Autodesk Inventor part; units mm, degrees
(part 2 of 3)
  arc A175 (-37.2013, 68.5038) -> (-37.3635, 68.3097) centre (-36.1751, 67.4815) ccw
  line L41 (-37.3635, 68.3097) -> (-37.4284, 68.2167)
  line L42 (-37.4284, 68.2167) -> (-36.811, 67.6337)
  line L43 (-36.811, 67.6337) -> (-36.1936, 67.0508)
  line L44 (-36.1936, 67.0508) -> (-36.0674, 67.2032)
  arc A176 (-35.5543, 67.7509) -> (-36.0674, 67.2032) centre (-31.3354, 63.2844) ccw
  arc A177 (-34.9902, 68.2176) -> (-35.5543, 67.7509) centre (-31.7324, 63.7046) ccw
  arc A178 (-34.3783, 68.5998) -> (-34.9902, 68.2176) centre (-31.8294, 63.839) ccw
  arc A179 (-33.7228, 68.8958) -> (-34.3783, 68.5998) centre (-31.86, 63.8962) ccw
  arc A180 (-32.0401, 69.2429) -> (-33.7228, 68.8958) centre (-31.7577, 63.6217) ccw
  arc A181 (-30.349, 69.0602) -> (-32.0401, 69.2429) centre (-31.7686, 63.8379) ccw
  arc A182 (-28.7916, 68.3601) -> (-30.349, 69.0602) centre (-31.7807, 63.7933) ccw
  arc A183 (-27.4976, 67.2036) -> (-28.7916, 68.3601) centre (-31.976, 63.4949) ccw
  line L45 (-27.4976, 67.2036) -> (-27.3717, 67.0515)
  line L46 (-27.3717, 67.0515) -> (-26.7547, 67.6348)
  line L47 (-26.7547, 67.6348) -> (-26.1378, 68.218)
  line L48 (-26.1378, 68.218) -> (-26.2023, 68.3104)
  arc A184 (-26.2023, 68.3104) -> (-26.2473, 68.3665) centre (-26.6433, 68.0026) ccw
  arc A185 (-26.2473, 68.3665) -> (-26.3703, 68.4988) centre (-37.3359, 58.178) ccw
  arc A186 (-26.3703, 68.4988) -> (-26.5193, 68.6547) centre (-36.4537, 59.0082) ccw
  arc A187 (-26.5193, 68.6547) -> (-26.6838, 68.822) centre (-40.4031, 55.1733) ccw
  arc A188 (-26.6838, 68.822) -> (-27.1502, 69.256) centre (-32.5321, 63.0037) ccw
  arc A189 (-27.1502, 69.256) -> (-27.6227, 69.6261) centre (-31.3885, 64.3323) ccw
  arc A190 (-27.6227, 69.6261) -> (-28.1264, 69.9504) centre (-31.375, 64.3513) ccw
  arc A191 (-28.1264, 69.9504) -> (-28.687, 70.247) centre (-32.2022, 62.9256) ccw
  arc A192 (-28.687, 70.247) -> (-29.244, 70.4848) centre (-31.6549, 64.0655) ccw
  arc A193 (-29.244, 70.4848) -> (-29.8311, 70.6779) centre (-31.8578, 63.5254) ccw
  arc A194 (-29.8311, 70.6779) -> (-30.4329, 70.8217) centre (-31.863, 63.5069) ccw
  arc A195 (-30.4329, 70.8217) -> (-31.0343, 70.9122) centre (-31.7664, 64.0012) ccw
  arc A196 (-31.0343, 70.9122) -> (-31.3562, 70.9333) centre (-31.4614, 66.8798) ccw
  arc A197 (-31.3562, 70.9333) -> (-31.8226, 70.939) centre (-31.7967, 53.9604) ccw
  arc A198 (-31.8226, 70.939) -> (-32.2848, 70.9321) centre (-31.7963, 53.7113) ccw
  arc A199 (-32.2848, 70.9321) -> (-32.5832, 70.9098) centre (-32.1934, 67.7089) ccw
  arc A200 (-32.0904, 68.184) -> (-32.8869, 68.0454) centre (-31.5556, 62.7535) ccw
  arc A201 (-32.8869, 68.0454) -> (-33.6094, 67.7947) centre (-31.8192, 63.8013) ccw
  arc A202 (-33.6094, 67.7947) -> (-34.2629, 67.4283) centre (-31.8964, 63.9735) ccw
  arc A203 (-34.2629, 67.4283) -> (-34.854, 66.9451) centre (-31.7132, 63.7061) ccw
  arc A204 (-34.854, 66.9451) -> (-35.0438, 66.7534) centre (-30.2573, 62.2047) ccw
  arc A205 (-35.0438, 66.7534) -> (-35.2248, 66.5549) centre (-30.3374, 62.2808) ccw
  arc A206 (-35.2248, 66.5549) -> (-35.3825, 66.371) centre (-25.9009, 58.401) ccw
  arc A207 (-35.3825, 66.371) -> (-35.4014, 66.3193) centre (-35.321, 66.3193) ccw
  arc A208 (-35.4014, 66.3193) -> (-35.3918, 66.297) centre (-35.3708, 66.3193) ccw
  arc A209 (-35.3918, 66.297) -> (-34.7975, 65.7374) centre (1437.4655, 1629.9498) ccw
  arc A210 (-34.7975, 65.7374) -> (-34.211, 65.1858) centre (719.0411, 866.6564) ccw
  arc A211 (-34.211, 65.1858) -> (-34.1695, 65.1598) centre (-34.1239, 65.2785) ccw
  arc A212 (-34.1695, 65.1598) -> (-34.1552, 65.163) centre (-34.1647, 65.1721) ccw
  arc A213 (-34.1552, 65.163) -> (-34.1121, 65.2103) centre (-35.4224, 66.3612) ccw
  arc A214 (-34.1121, 65.2103) -> (-34.062, 65.2709) centre (-35.0787, 66.0593) ccw
  arc A215 (-34.062, 65.2709) -> (-34.0071, 65.3446) centre (-35.9526, 66.7371) ccw
  arc A216 (-33.6777, 65.7235) -> (-34.0071, 65.3446) centre (-31.8426, 63.7953) ccw
  arc A217 (-33.2793, 66.0389) -> (-33.6777, 65.7235) centre (-31.7523, 63.7004) ccw
  arc A218 (-32.8278, 66.2785) -> (-33.2793, 66.0389) centre (-31.7341, 63.6725) ccw
  arc A219 (-32.3411, 66.4325) -> (-32.8278, 66.2785) centre (-31.7393, 63.6849) ccw
  arc A220 (-32.0556, 66.4702) -> (-32.3411, 66.4325) centre (-31.9755, 64.7634) ccw
  arc A221 (-31.6858, 66.4725) -> (-32.0556, 66.4702) centre (-31.8417, 61.911) ccw
  arc A222 (-31.3168, 66.4449) -> (-31.6858, 66.4725) centre (-31.8418, 61.9075) ccw
  arc A223 (-31.0333, 66.3878) -> (-31.3168, 66.4449) centre (-31.5158, 64.7246) ccw
  arc A224 (-30.6006, 66.2181) -> (-31.0333, 66.3878) centre (-31.743, 63.9414) ccw
  arc A225 (-30.1846, 65.966) -> (-30.6006, 66.2181) centre (-31.9687, 63.4917) ccw
  arc A226 (-29.8154, 65.652) -> (-30.1846, 65.966) centre (-31.9569, 63.5081) ccw
  arc A227 (-29.5219, 65.298) -> (-29.8154, 65.652) centre (-31.554, 63.9115) ccw
  arc A228 (-29.5219, 65.298) -> (-29.4814, 65.242) centre (-28.4557, 66.0255) ccw
  arc A229 (-29.4814, 65.242) -> (-29.4433, 65.1963) centre (-28.9168, 65.6733) ccw
  arc A230 (-29.4433, 65.1963) -> (-29.4105, 65.1624) centre (-28.9075, 65.6817) ccw
  arc A231 (-29.4105, 65.1624) -> (-29.3963, 65.1594) centre (-29.4011, 65.1721) ccw
  arc A232 (-29.3963, 65.1594) -> (-29.3562, 65.1846) centre (-29.44, 65.2739) ccw
  arc A233 (-29.3562, 65.1846) -> (-28.7682, 65.7366) centre (-840.8345, 930.1184) ccw
  arc A234 (-28.7682, 65.7366) -> (-28.1727, 66.2963) centre (-1600.6595, 1738.8944) ccw
  arc A235 (-28.1727, 66.2963) -> (-28.1634, 66.3178) centre (-28.1929, 66.3178) ccw
  arc A236 (-28.1634, 66.3178) -> (-28.1663, 66.3266) centre (-28.1782, 66.3178) ccw
  arc A237 (-28.1663, 66.3266) -> (-28.2084, 66.3834) centre (-38.1616, 58.9544) ccw
  arc A238 (-28.2084, 66.3834) -> (-28.258, 66.4485) centre (-31.6783, 63.7935) ccw
  arc A239 (-28.258, 66.4485) -> (-28.3168, 66.5233) centre (-34.5032, 61.6007) ccw
  arc A240 (-28.3168, 66.5233) -> (-28.6224, 66.8616) centre (-31.1638, 64.2579) ccw
  arc A241 (-28.6224, 66.8616) -> (-29.0001, 67.1976) centre (-32.4574, 62.9327) ccw
  arc A242 (-29.0001, 67.1976) -> (-29.4081, 67.4984) centre (-32.4734, 62.9129) ccw
  arc A243 (-29.4081, 67.4984) -> (-29.8056, 67.7302) centre (-31.4926, 64.3801) ccw
  arc A244 (-29.8056, 67.7302) -> (-30.0614, 67.8432) centre (-31.0503, 65.2584) ccw
  arc A245 (-30.0614, 67.8432) -> (-30.3939, 67.9608) centre (-32.5323, 61.3851) ccw
  arc A246 (-30.3939, 67.9608) -> (-30.7335, 68.0617) centre (-32.5419, 61.3556) ccw
  arc A247 (-30.7335, 68.0617) -> (-31.0124, 68.1226) centre (-31.5028, 65.209) ccw
  arc A248 (-31.0124, 68.1226) -> (-31.2629, 68.1554) centre (-31.5838, 64.7277) ccw
  arc A249 (-31.2629, 68.1554) -> (-31.5824, 68.1794) centre (-32.0821, 59.4058) ccw
  arc A250 (-31.5824, 68.1794) -> (-31.8907, 68.1916) centre (-32.0866, 59.3265) ccw
  arc A251 (-31.8907, 68.1916) -> (-32.0904, 68.184) centre (-31.9274, 66.5294) ccw
  arc A252 (-32.1366, 65.3865) -> (-32.5528, 65.1937) centre (-31.7549, 64.017) ccw
  arc A253 (-32.5528, 65.1937) -> (-32.8895, 64.8772) centre (-31.7317, 63.9828) ccw
  arc A254 (-32.8895, 64.8772) -> (-33.1084, 64.4743) centre (-31.7513, 63.998) ccw
  arc A255 (-33.1084, 64.4743) -> (-33.1834, 64.0313) centre (-31.8538, 64.0339) ccw
  arc A256 (-33.1834, 64.0313) -> (-33.0398, 63.4203) centre (-31.8003, 64.0341) ccw
  arc A257 (-33.0398, 63.4203) -> (-32.6401, 62.9292) centre (-31.759, 64.0545) ccw
  arc A258 (-32.6401, 62.9292) -> (-32.07, 62.6613) centre (-31.7694, 64.0412) ccw
  arc A259 (-32.07, 62.6613) -> (-31.4495, 62.6738) centre (-31.7859, 63.9654) ccw
  arc A260 (-31.4495, 62.6738) -> (-31.0909, 62.817) centre (-31.839, 64.1692) ccw
  arc A261 (-31.0909, 62.817) -> (-30.7938, 63.0407) centre (-31.7358, 63.9827) ccw
  arc A262 (-30.7938, 63.0407) -> (-30.5702, 63.3378) centre (-31.7358, 63.9827) ccw
  arc A263 (-30.5702, 63.3378) -> (-30.4269, 63.6964) centre (-31.9224, 64.0859) ccw
  arc A264 (-30.4269, 63.6964) -> (-30.4151, 64.3239) centre (-31.7256, 64.0347) ccw
  arc A265 (-30.4151, 64.3239) -> (-30.6888, 64.8964) centre (-31.7815, 64.0223) ccw
  arc A266 (-30.6888, 64.8964) -> (-31.1897, 65.2927) centre (-31.7983, 64.0089) ccw
  arc A267 (-31.1897, 65.2927) -> (-31.8119, 65.4279) centre (-31.7912, 64.0239) ccw
  arc A268 (-31.8119, 65.4279) -> (-31.8933, 65.424) centre (-31.7935, 64.1823) ccw
  arc A269 (-31.8933, 65.424) -> (-31.984, 65.4146) centre (-31.7364, 63.4723) ccw
  arc A270 (-31.984, 65.4146) -> (-32.0702, 65.4015) centre (-31.75, 63.5786) ccw
  arc A271 (-32.0702, 65.4015) -> (-32.1366, 65.3865) centre (-31.95, 64.7171) ccw
  arc A272 (-30.9168, 15.2189) -> (-29.3545, 15.4735) centre (-31.794, 25.5192) ccw
  arc A273 (-29.3545, 15.4735) -> (-27.8672, 15.9622) centre (-31.6889, 25.0867) ccw
  arc A274 (-27.8672, 15.9622) -> (-26.477, 16.6788) centre (-31.6817, 25.0694) ccw
  arc A275 (-26.477, 16.6788) -> (-25.2034, 17.6119) centre (-31.8789, 25.3873) ccw
  arc A276 (-25.2034, 17.6119) -> (-24.9272, 17.861) centre (-30.1736, 23.401) ccw
  arc A277 (-24.9272, 17.861) -> (-24.6106, 18.1697) centre (-35.3442, 28.861) ccw
  arc A278 (-24.6106, 18.1697) -> (-24.3181, 18.4718) centre (-35.0871, 28.6048) ccw
  arc A279 (-24.3181, 18.4718) -> (-24.1302, 18.6893) centre (-26.7779, 20.7864) ccw
  line L49 (-24.1302, 18.6893) -> (-24.0364, 18.8078)
  line L50 (-24.0364, 18.8078) -> (-24.6584, 19.3804)
  line L51 (-24.6584, 19.3804) -> (-25.2804, 19.9531)
  line L52 (-25.2804, 19.9531) -> (-25.4467, 19.7631)
  arc A280 (-26.4222, 18.8133) -> (-25.4467, 19.7631) centre (-31.8805, 25.3952) ccw
  arc A281 (-27.5365, 18.0299) -> (-26.4222, 18.8133) centre (-31.8906, 25.4074) ccw
  arc A282 (-28.7501, 17.4395) -> (-27.5365, 18.0299) centre (-31.81, 25.2709) ccw
  arc A283 (-30.0209, 17.0635) -> (-28.7501, 17.4395) centre (-31.5963, 24.724) ccw
  arc A284 (-30.8588, 16.936) -> (-30.0209, 17.0635) centre (-31.6693, 25.079) ccw
  arc A285 (-31.7176, 16.8933) -> (-30.8588, 16.936) centre (-31.7176, 25.5643) ccw
  arc A286 (-32.5765, 16.936) -> (-31.7176, 16.8933) centre (-31.7176, 25.5643) ccw
  arc A287 (-33.4143, 17.0635) -> (-32.5765, 16.936) centre (-31.7659, 25.079) ccw
  arc A288 (-34.6853, 17.439) -> (-33.4143, 17.0635) centre (-31.8322, 24.7569) ccw
  arc A289 (-35.8956, 18.0273) -> (-34.6853, 17.439) centre (-31.653, 25.2164) ccw
  arc A290 (-37.0081, 18.8098) -> (-35.8956, 18.0273) centre (-31.5598, 25.3743) ccw
  arc A291 (-37.9883, 19.7628) -> (-37.0081, 18.8098) centre (-31.4492, 25.5076) ccw
  line L53 (-37.9883, 19.7628) -> (-38.1548, 19.9524)
  line L54 (-38.1548, 19.9524) -> (-38.7772, 19.3805)
  line L55 (-38.7772, 19.3805) -> (-39.3995, 18.8086)
  line L56 (-39.3995, 18.8086) -> (-39.3018, 18.6827)
  arc A292 (-39.3018, 18.6827) -> (-39.0982, 18.4502) centre (-37.247, 20.277) ccw
  arc A293 (-39.0982, 18.4502) -> (-38.6947, 18.0503) centre (-20.8164, 36.4914) ccw
  arc A294 (-38.6947, 18.0503) -> (-38.2739, 17.6523) centre (-22.4071, 34.8506) ccw
  arc A295 (-38.2739, 17.6523) -> (-37.97, 17.3915) centre (-34.4969, 21.7463) ccw
  arc A296 (-37.97, 17.3915) -> (-36.7254, 16.5398) centre (-31.5357, 25.4591) ccw
  arc A297 (-36.7254, 16.5398) -> (-35.3826, 15.8887) centre (-31.7481, 25.0939) ccw
  arc A298 (-35.3826, 15.8887) -> (-33.9556, 15.4462) centre (-31.7395, 25.1157) ccw
  arc A299 (-33.9556, 15.4462) -> (-32.4601, 15.2161) centre (-31.6251, 25.6151) ccw
  arc A300 (-32.4601, 15.2161) -> (-32.0962, 15.1956) centre (-31.8541, 22.7628) ccw
  arc A301 (-32.0962, 15.1956) -> (-31.6859, 15.1895) centre (-31.708, 27.3292) ccw
  arc A302 (-31.6859, 15.1895) -> (-31.2769, 15.1971) centre (-31.7079, 27.2755) ccw
  arc A303 (-31.2769, 15.1971) -> (-30.9168, 15.2189) centre (-31.538, 22.5135) ccw
  arc A304 (-30.9168, 17.9902) -> (-29.9577, 18.169) centre (-31.8527, 25.6751) ccw
  arc A305 (-29.9577, 18.169) -> (-29.0477, 18.4646) centre (-31.7105, 25.112) ccw
  arc A306 (-29.0477, 18.4646) -> (-28.1832, 18.8798) centre (-31.724, 25.1455) ccw
  arc A307 (-28.1832, 18.8798) -> (-27.3594, 19.4152) centre (-32.0807, 25.7768) ccw
  arc A308 (-27.3594, 19.4152) -> (-27.0939, 19.6338) centre (-29.3965, 22.1601) ccw
  arc A309 (-27.0939, 19.6338) -> (-26.6906, 20.0113) centre (-41.2454, 35.1596) ccw
  arc A310 (-26.6906, 20.0113) -> (-26.2987, 20.3962) centre (-44.0969, 38.1275) ccw
  arc A311 (-26.2987, 20.3962) -> (-26.1365, 20.5903) centre (-27.3249, 21.4185) ccw
  line L57 (-26.1365, 20.5903) -> (-26.0716, 20.6833)
  line L58 (-26.0716, 20.6833) -> (-26.689, 21.2663)
  line L59 (-26.689, 21.2663) -> (-27.3064, 21.8492)
  line L60 (-27.3064, 21.8492) -> (-27.4326, 21.6968)
  arc A312 (-27.9457, 21.1491) -> (-27.4326, 21.6968) centre (-32.1646, 25.6156) ccw
  arc A313 (-28.5098, 20.6824) -> (-27.9457, 21.1491) centre (-31.7676, 25.1954) ccw
  arc A314 (-29.1217, 20.3002) -> (-28.5098, 20.6824) centre (-31.6706, 25.061) ccw
  arc A315 (-29.7772, 20.0042) -> (-29.1217, 20.3002) centre (-31.64, 25.0038) ccw
  arc A316 (-31.4599, 19.6571) -> (-29.7772, 20.0042) centre (-31.7423, 25.2783) ccw
  arc A317 (-33.151, 19.8398) -> (-31.4599, 19.6571) centre (-31.7314, 25.0621) ccw
  arc A318 (-34.7084, 20.5399) -> (-33.151, 19.8398) centre (-31.7193, 25.1067) ccw
  arc A319 (-36.0024, 21.6964) -> (-34.7084, 20.5399) centre (-31.524, 25.4051) ccw
  line L61 (-36.0024, 21.6964) -> (-36.1283, 21.8485)
  line L62 (-36.1283, 21.8485) -> (-36.7453, 21.2652)
  line L63 (-36.7453, 21.2652) -> (-37.3622, 20.682)
  line L64 (-37.3622, 20.682) -> (-37.2977, 20.5896)
  arc A320 (-37.2977, 20.5896) -> (-37.2527, 20.5335) centre (-36.8567, 20.8974) ccw
  arc A321 (-37.2527, 20.5335) -> (-37.1297, 20.4012) centre (-26.1641, 30.722) ccw
  arc A322 (-37.1297, 20.4012) -> (-36.9807, 20.2453) centre (-27.0463, 29.8918) ccw
  arc A323 (-36.9807, 20.2453) -> (-36.8162, 20.078) centre (-23.0969, 33.7267) ccw
  arc A324 (-36.8162, 20.078) -> (-36.3498, 19.644) centre (-30.9679, 25.8963) ccw
  arc A325 (-36.3498, 19.644) -> (-35.8773, 19.2739) centre (-32.1115, 24.5677) ccw
  arc A326 (-35.8773, 19.2739) -> (-35.3736, 18.9496) centre (-32.125, 24.5487) ccw
  arc A327 (-35.3736, 18.9496) -> (-34.813, 18.653) centre (-31.2978, 25.9744) ccw
  arc A328 (-34.813, 18.653) -> (-34.256, 18.4152) centre (-31.8451, 24.8345) ccw
  arc A329 (-34.256, 18.4152) -> (-33.6689, 18.2221) centre (-31.6422, 25.3746) ccw
  arc A330 (-33.6689, 18.2221) -> (-33.0671, 18.0783) centre (-31.637, 25.3931) ccw
  arc A331 (-33.0671, 18.0783) -> (-32.4657, 17.9878) centre (-31.7336, 24.8988) ccw
  arc A332 (-32.4657, 17.9878) -> (-32.1438, 17.9667) centre (-32.0386, 22.0202) ccw
  arc A333 (-32.1438, 17.9667) -> (-31.6774, 17.961) centre (-31.7033, 34.9396) ccw
  arc A334 (-31.6774, 17.961) -> (-31.2152, 17.9679) centre (-31.7037, 35.1887) ccw
  arc A335 (-31.2152, 17.9679) -> (-30.9168, 17.9902) centre (-31.3066, 21.1911) ccw
  arc A336 (-31.4096, 20.716) -> (-30.6131, 20.8546) centre (-31.9444, 26.1465) ccw
  arc A337 (-30.6131, 20.8546) -> (-29.8906, 21.1053) centre (-31.6808, 25.0987) ccw
  arc A338 (-29.8906, 21.1053) -> (-29.2371, 21.4717) centre (-31.6036, 24.9265) ccw
  arc A339 (-29.2371, 21.4717) -> (-28.646, 21.9549) centre (-31.7868, 25.1939) ccw
  arc A340 (-28.646, 21.9549) -> (-28.4562, 22.1466) centre (-33.2427, 26.6953) ccw
  arc A341 (-28.4562, 22.1466) -> (-28.2752, 22.3451) centre (-33.1626, 26.6192) ccw
  arc A342 (-28.2752, 22.3451) -> (-28.1175, 22.529) centre (-37.5991, 30.499) ccw
  arc A343 (-28.1175, 22.529) -> (-28.0986, 22.5807) centre (-28.179, 22.5807) ccw
  arc A344 (-28.0986, 22.5807) -> (-28.1082, 22.603) centre (-28.1292, 22.5807) ccw
  arc A345 (-28.1082, 22.603) -> (-28.7025, 23.1626) centre (-1500.9655, -1541.0498) ccw
  arc A346 (-28.7025, 23.1626) -> (-29.289, 23.7142) centre (-782.5411, -777.7564) ccw
  arc A347 (-29.289, 23.7142) -> (-29.3305, 23.7402) centre (-29.3761, 23.6215) ccw
  arc A348 (-29.3305, 23.7402) -> (-29.3448, 23.737) centre (-29.3353, 23.7279) ccw
  arc A349 (-29.3448, 23.737) -> (-29.3879, 23.6897) centre (-28.0776, 22.5388) ccw
  arc A350 (-29.3879, 23.6897) -> (-29.438, 23.6291) centre (-28.4213, 22.8407) ccw
  arc A351 (-29.438, 23.6291) -> (-29.4929, 23.5554) centre (-27.5474, 22.1629) ccw
  arc A352 (-29.8223, 23.1765) -> (-29.4929, 23.5554) centre (-31.6574, 25.1047) ccw
  arc A353 (-30.2207, 22.8611) -> (-29.8223, 23.1765) centre (-31.7477, 25.1996) ccw
  arc A354 (-30.6722, 22.6215) -> (-30.2207, 22.8611) centre (-31.7659, 25.2275) ccw
  arc A355 (-31.1589, 22.4675) -> (-30.6722, 22.6215) centre (-31.7607, 25.2151) ccw
  arc A356 (-31.4444, 22.4298) -> (-31.1589, 22.4675) centre (-31.5245, 24.1366) ccw
  arc A357 (-31.8142, 22.4275) -> (-31.4444, 22.4298) centre (-31.6583, 26.989) ccw
  arc A358 (-32.1832, 22.4551) -> (-31.8142, 22.4275) centre (-31.6582, 26.9925) ccw
  arc A359 (-32.4667, 22.5122) -> (-32.1832, 22.4551) centre (-31.9842, 24.1754) ccw
  arc A360 (-32.8994, 22.6819) -> (-32.4667, 22.5122) centre (-31.757, 24.9586) ccw
  arc A361 (-33.3154, 22.934) -> (-32.8994, 22.6819) centre (-31.5313, 25.4083) ccw
  arc A362 (-33.6846, 23.248) -> (-33.3154, 22.934) centre (-31.5431, 25.3919) ccw
  arc A363 (-33.9781, 23.602) -> (-33.6846, 23.248) centre (-31.946, 24.9885) ccw
  arc A364 (-33.9781, 23.602) -> (-34.0186, 23.658) centre (-35.0443, 22.8745) ccw
  arc A365 (-34.0186, 23.658) -> (-34.0567, 23.7037) centre (-34.5832, 23.2267) ccw
  arc A366 (-34.0567, 23.7037) -> (-34.0895, 23.7376) centre (-34.5925, 23.2183) ccw
  arc A367 (-34.0895, 23.7376) -> (-34.1037, 23.7406) centre (-34.0989, 23.7279) ccw
  arc A368 (-34.1037, 23.7406) -> (-34.1438, 23.7154) centre (-34.06, 23.6261) ccw
  arc A369 (-34.1438, 23.7154) -> (-34.7318, 23.1634) centre (777.3345, -841.2184) ccw
  arc A370 (-34.7318, 23.1634) -> (-35.3273, 22.6037) centre (1537.1595, -1649.9944) ccw
  arc A371 (-35.3273, 22.6037) -> (-35.3366, 22.5822) centre (-35.3071, 22.5822) ccw
  arc A372 (-35.3366, 22.5822) -> (-35.3337, 22.5734) centre (-35.3218, 22.5822) ccw
  arc A373 (-35.3337, 22.5734) -> (-35.2916, 22.5166) centre (-25.3384, 29.9456) ccw
  arc A374 (-35.2916, 22.5166) -> (-35.242, 22.4515) centre (-31.8217, 25.1065) ccw
  arc A375 (-35.242, 22.4515) -> (-35.1832, 22.3767) centre (-28.9968, 27.2993) ccw
  arc A376 (-35.1832, 22.3767) -> (-34.8776, 22.0384) centre (-32.3362, 24.6421) ccw
  arc A377 (-34.8776, 22.0384) -> (-34.4999, 21.7024) centre (-31.0426, 25.9673) ccw
  arc A378 (-34.4999, 21.7024) -> (-34.0919, 21.4016) centre (-31.0266, 25.9871) ccw
  arc A379 (-34.0919, 21.4016) -> (-33.6944, 21.1698) centre (-32.0074, 24.5199) ccw
  arc A380 (-33.6944, 21.1698) -> (-33.4386, 21.0568) centre (-32.4497, 23.6416) ccw
  arc A381 (-33.4386, 21.0568) -> (-33.1061, 20.9392) centre (-30.9677, 27.5149) ccw
  arc A382 (-33.1061, 20.9392) -> (-32.7665, 20.8383) centre (-30.9581, 27.5444) ccw
  arc A383 (-32.7665, 20.8383) -> (-32.4876, 20.7774) centre (-31.9972, 23.691) ccw
  arc A384 (-32.4876, 20.7774) -> (-32.2371, 20.7446) centre (-31.9162, 24.1723) ccw
  arc A385 (-32.2371, 20.7446) -> (-31.9176, 20.7206) centre (-31.4179, 29.4942) ccw
  arc A386 (-31.9176, 20.7206) -> (-31.6093, 20.7084) centre (-31.4134, 29.5735) ccw
  arc A387 (-31.6093, 20.7084) -> (-31.4096, 20.716) centre (-31.5726, 22.3706) ccw
  arc A388 (-31.3634, 23.5135) -> (-30.9472, 23.7063) centre (-31.7451, 24.883) ccw
  arc A389 (-30.9472, 23.7063) -> (-30.6105, 24.0228) centre (-31.7683, 24.9172) ccw
  arc A390 (-30.6105, 24.0228) -> (-30.3916, 24.4257) centre (-31.7487, 24.902) ccw
  arc A391 (-30.3916, 24.4257) -> (-30.3166, 24.8687) centre (-31.6462, 24.8661) ccw
  arc A392 (-30.3166, 24.8687) -> (-30.4602, 25.4797) centre (-31.6997, 24.8659) ccw
  arc A393 (-30.4602, 25.4797) -> (-30.8599, 25.9708) centre (-31.741, 24.8455) ccw
  arc A394 (-30.8599, 25.9708) -> (-31.43, 26.2387) centre (-31.7306, 24.8588) ccw
  arc A395 (-31.43, 26.2387) -> (-32.0505, 26.2262) centre (-31.7141, 24.9346) ccw
  arc A396 (-32.0505, 26.2262) -> (-32.4091, 26.083) centre (-31.661, 24.7308) ccw
  arc A397 (-32.4091, 26.083) -> (-32.7062, 25.8593) centre (-31.7642, 24.9173) ccw
  arc A398 (-32.7062, 25.8593) -> (-32.9298, 25.5622) centre (-31.7642, 24.9173) ccw
  arc A399 (-32.9298, 25.5622) -> (-33.0731, 25.2036) centre (-31.5776, 24.8141) ccw
  arc A400 (-33.0731, 25.2036) -> (-33.0849, 24.5761) centre (-31.7744, 24.8653) ccw
  arc A401 (-33.0849, 24.5761) -> (-32.8112, 24.0036) centre (-31.7185, 24.8777) ccw
  arc A402 (-32.8112, 24.0036) -> (-32.3103, 23.6073) centre (-31.7017, 24.8911) ccw
  arc A403 (-32.3103, 23.6073) -> (-31.6881, 23.4721) centre (-31.7088, 24.8761) ccw
  arc A404 (-31.6881, 23.4721) -> (-31.6067, 23.476) centre (-31.7065, 24.7177) ccw
  arc A405 (-31.6067, 23.476) -> (-31.516, 23.4854) centre (-31.7636, 25.4277) ccw
  arc A406 (-31.516, 23.4854) -> (-31.4298, 23.4985) centre (-31.75, 25.3214) ccw
  arc A407 (-31.4298, 23.4985) -> (-31.3634, 23.5135) centre (-31.55, 24.1829) ccw
  arc A408 (-54.2587, 71.8195) -> (-55.2164, 71.6633) centre (-53.721, 65.5053) ccw
  arc A409 (-55.2164, 71.6633) -> (-56.1281, 71.3638) centre (-53.7854, 65.7705) ccw
  arc A410 (-56.1281, 71.3638) -> (-56.9803, 70.9245) centre (-53.7898, 65.7811) ccw
  arc A411 (-56.9803, 70.9245) -> (-57.761, 70.3525) centre (-53.6689, 65.5862) ccw
  arc A412 (-57.761, 70.3525) -> (-57.9303, 70.1998) centre (-54.7143, 66.8038) ccw
  arc A413 (-57.9303, 70.1998) -> (-58.1244, 70.0106) centre (-51.5447, 63.4568) ccw
  arc A414 (-58.1244, 70.0106) -> (-58.3037, 69.8254) centre (-51.7023, 63.6139) ccw
  arc A415 (-58.3037, 69.8254) -> (-58.4189, 69.6921) centre (-56.7958, 68.4066) ccw
  line L65 (-58.4189, 69.6921) -> (-58.4764, 69.6194)
  line L66 (-58.4764, 69.6194) -> (-58.0951, 69.2684)
  line L67 (-58.0951, 69.2684) -> (-57.7138, 68.9174)
  line L68 (-57.7138, 68.9174) -> (-57.6118, 69.0338)
  arc A416 (-57.0139, 69.616) -> (-57.6118, 69.0338) centre (-53.6679, 65.5813) ccw
  arc A417 (-56.3308, 70.0963) -> (-57.0139, 69.616) centre (-53.6618, 65.5739) ccw
  arc A418 (-55.5869, 70.4582) -> (-56.3308, 70.0963) centre (-53.7111, 65.6576) ccw
  arc A419 (-54.8079, 70.6887) -> (-55.5869, 70.4582) centre (-53.8421, 65.9928) ccw
  arc A420 (-54.2943, 70.7669) -> (-54.8079, 70.6887) centre (-53.7974, 65.7752) ccw
  arc A421 (-53.7678, 70.793) -> (-54.2943, 70.7669) centre (-53.7678, 65.4777) ccw
  arc A422 (-53.2413, 70.7669) -> (-53.7678, 70.793) centre (-53.7678, 65.4777) ccw
  arc A423 (-52.7277, 70.6887) -> (-53.2413, 70.7669) centre (-53.7382, 65.7752) ccw
  arc A424 (-51.9486, 70.4585) -> (-52.7277, 70.6887) centre (-53.6976, 65.9726) ccw
  arc A425 (-51.2067, 70.0979) -> (-51.9486, 70.4585) centre (-53.8074, 65.6909) ccw
  arc A426 (-50.5247, 69.6182) -> (-51.2067, 70.0979) centre (-53.8645, 65.5942) ccw
  arc A427 (-49.9239, 69.034) -> (-50.5247, 69.6182) centre (-53.9323, 65.5125) ccw
  line L69 (-49.9239, 69.034) -> (-49.8218, 68.9178)
  line L70 (-49.8218, 68.9178) -> (-49.4403, 69.2684)
  line L71 (-49.4403, 69.2684) -> (-49.0588, 69.619)
  line L72 (-49.0588, 69.619) -> (-49.1187, 69.6961)
  arc A428 (-49.1187, 69.6961) -> (-49.2435, 69.8387) centre (-50.3783, 68.7188) ccw
  arc A429 (-49.2435, 69.8387) -> (-49.4908, 70.0838) centre (-60.4502, 58.7794) ccw
  arc A430 (-49.4908, 70.0838) -> (-49.7488, 70.3278) centre (-59.4752, 59.7852) ccw
  arc A431 (-49.7488, 70.3278) -> (-49.9351, 70.4876) centre (-52.0641, 67.8182) ccw
  arc A432 (-49.9351, 70.4876) -> (-50.698, 71.0097) centre (-53.8793, 65.5422) ccw
  arc A433 (-50.698, 71.0097) -> (-51.5212, 71.4089) centre (-53.7491, 65.766) ccw
  arc A434 (-51.5212, 71.4089) -> (-52.3959, 71.6801) centre (-53.7544, 65.7527) ccw
  arc A435 (-52.3959, 71.6801) -> (-53.3127, 71.8212) centre (-53.8245, 65.4466) ccw
  arc A436 (-53.3127, 71.8212) -> (-53.5357, 71.8337) centre (-53.6841, 67.195) ccw
  arc A437 (-53.5357, 71.8337) -> (-53.7872, 71.8375) centre (-53.7737, 64.3958) ccw
  arc A438 (-53.7872, 71.8375) -> (-54.0379, 71.8328) centre (-53.7737, 64.4287) ccw
  arc A439 (-54.0379, 71.8328) -> (-54.2587, 71.8195) centre (-53.8779, 67.3479) ccw
  arc A440 (-54.2587, 70.1206) -> (-54.8466, 70.011) centre (-53.685, 65.4098) ccw
  arc A441 (-54.8466, 70.011) -> (-55.4044, 69.8298) centre (-53.7721, 65.755) ccw
  arc A442 (-55.4044, 69.8298) -> (-55.9344, 69.5753) centre (-53.7639, 65.7344) ccw
  arc A443 (-55.9344, 69.5753) -> (-56.4394, 69.2471) centre (-53.5452, 65.3475) ccw
  arc A444 (-56.4394, 69.2471) -> (-56.6021, 69.1131) centre (-55.1906, 67.5645) ccw
  arc A445 (-56.6021, 69.1131) -> (-56.8494, 68.8817) centre (-47.9272, 59.5958) ccw
  arc A446 (-56.8494, 68.8817) -> (-57.0896, 68.6458) centre (-46.1793, 57.7765) ccw
  arc A447 (-57.0896, 68.6458) -> (-57.189, 68.5268) centre (-56.4605, 68.0191) ccw
  line L73 (-57.189, 68.5268) -> (-57.2288, 68.4697)
  line L74 (-57.2288, 68.4697) -> (-56.8503, 68.1124)
  line L75 (-56.8503, 68.1124) -> (-56.4719, 67.7551)
  line L76 (-56.4719, 67.7551) -> (-56.3945, 67.8485)
  arc A448 (-56.08, 68.1842) -> (-56.3945, 67.8485) centre (-53.4938, 65.4462) ccw
  arc A449 (-55.7342, 68.4703) -> (-56.08, 68.1842) centre (-53.7371, 65.7039) ccw
  arc A450 (-55.3591, 68.7046) -> (-55.7342, 68.4703) centre (-53.7966, 65.7862) ccw
  arc A451 (-54.9572, 68.886) -> (-55.3591, 68.7046) centre (-53.8154, 65.8213) ccw
  arc A452 (-53.9257, 69.0988) -> (-54.9572, 68.886) centre (-53.7527, 65.653) ccw
  arc A453 (-52.8891, 68.9868) -> (-53.9257, 69.0988) centre (-53.7593, 65.7856) ccw
  arc A454 (-51.9344, 68.5576) -> (-52.8891, 68.9868) centre (-53.7667, 65.7582) ccw
  arc A455 (-51.1412, 67.8487) -> (-51.9344, 68.5576) centre (-53.8865, 65.5753) ccw
  line L77 (-51.1412, 67.8487) -> (-51.064, 67.7555)
  line L78 (-51.064, 67.7555) -> (-50.6858, 68.113)
  line L79 (-50.6858, 68.113) -> (-50.3077, 68.4706)
  line L80 (-50.3077, 68.4706) -> (-50.3472, 68.5272)
  arc A456 (-50.3472, 68.5272) -> (-50.3748, 68.5616) centre (-50.6176, 68.3385) ccw
  arc A457 (-50.3748, 68.5616) -> (-50.4502, 68.6427) centre (-57.1721, 62.316) ccw
  arc A458 (-50.4502, 68.6427) -> (-50.5416, 68.7383) centre (-56.6313, 62.825) ccw
  arc A459 (-50.5416, 68.7383) -> (-50.6423, 68.8408) centre (-59.0523, 60.4741) ccw
  arc A460 (-50.6423, 68.8408) -> (-50.9283, 69.1069) centre (-54.2274, 65.2742) ccw
  arc A461 (-50.9283, 69.1069) -> (-51.2179, 69.3337) centre (-53.5264, 66.0886) ccw
  arc A462 (-51.2179, 69.3337) -> (-51.5267, 69.5325) centre (-53.5181, 66.1003) ccw
  arc A463 (-51.5267, 69.5325) -> (-51.8703, 69.7143) centre (-54.0251, 65.2263) ccw
  arc A464 (-51.8703, 69.7143) -> (-52.2117, 69.8601) centre (-53.6897, 65.9251) ccw
  arc A465 (-52.2117, 69.8601) -> (-52.5716, 69.9784) centre (-53.814, 65.594) ccw
  arc A466 (-52.5716, 69.9784) -> (-52.9406, 70.0666) centre (-53.8172, 65.5826) ccw
  arc A467 (-52.9406, 70.0666) -> (-53.3092, 70.1221) centre (-53.758, 65.8856) ccw
  arc A468 (-53.3092, 70.1221) -> (-53.5066, 70.1351) centre (-53.571, 67.6502) ccw
  arc A469 (-53.5066, 70.1351) -> (-53.7925, 70.1386) centre (-53.7766, 59.7306) ccw
  arc A470 (-53.7925, 70.1386) -> (-54.0758, 70.1343) centre (-53.7763, 59.5779) ccw
  arc A471 (-54.0758, 70.1343) -> (-54.2587, 70.1206) centre (-54.0197, 68.1585) ccw
  arc A472 (-53.9566, 68.4497) -> (-54.4448, 68.3648) centre (-53.6288, 65.1208) ccw
  arc A473 (-54.4448, 68.3648) -> (-54.8878, 68.2111) centre (-53.7904, 65.7631) ccw
  arc A474 (-54.8878, 68.2111) -> (-55.2884, 67.9865) centre (-53.8377, 65.8687) ccw
  arc A475 (-55.2884, 67.9865) -> (-55.6507, 67.6903) centre (-53.7254, 65.7048) ccw
  arc A476 (-55.6507, 67.6903) -> (-55.7671, 67.5728) centre (-52.8329, 64.7844) ccw
  arc A477 (-55.7671, 67.5728) -> (-55.878, 67.4511) centre (-52.882, 64.831) ccw
  arc A478 (-55.878, 67.4511) -> (-55.9747, 67.3383) centre (-50.1625, 62.4527) ccw
  arc A479 (-55.9747, 67.3383) -> (-55.9862, 67.3066) centre (-55.937, 67.3066) ccw
  arc A480 (-55.9862, 67.3066) -> (-55.9803, 67.293) centre (-55.9675, 67.3066) ccw
  arc A481 (-55.9803, 67.293) -> (-55.616, 66.95) centre (846.8811, 1025.8121) ccw
  arc A482 (-55.616, 66.95) -> (-55.2565, 66.6118) centre (406.487, 557.9133) ccw
  arc A483 (-55.2565, 66.6118) -> (-55.2311, 66.5959) centre (-55.2031, 66.6687) ccw
  arc A484 (-55.2311, 66.5959) -> (-55.2223, 66.5979) centre (-55.2282, 66.6034) ccw
  arc A485 (-55.2223, 66.5979) -> (-55.1959, 66.6269) centre (-55.9991, 67.3324) ccw
  arc A486 (-55.1959, 66.6269) -> (-55.1652, 66.664) centre (-55.7884, 67.1473) ccw
  arc A487 (-55.1652, 66.664) -> (-55.1316, 66.7092) centre (-56.3242, 67.5628) ccw
  arc A488 (-54.9296, 66.9414) -> (-55.1316, 66.7092) centre (-53.8047, 65.7595) ccw
  arc A489 (-54.6854, 67.1347) -> (-54.9296, 66.9414) centre (-53.7494, 65.7013) ccw
  arc A490 (-54.4086, 67.2816) -> (-54.6854, 67.1347) centre (-53.7382, 65.6842) ccw
  arc A491 (-54.1103, 67.376) -> (-54.4086, 67.2816) centre (-53.7414, 65.6918) ccw
  arc A492 (-53.9353, 67.3991) -> (-54.1103, 67.376) centre (-53.8862, 66.3529) ccw
  arc A493 (-53.7086, 67.4006) -> (-53.9353, 67.3991) centre (-53.8041, 64.6043) ccw
  arc A494 (-53.4824, 67.3837) -> (-53.7086, 67.4006) centre (-53.8042, 64.6022) ccw
  arc A495 (-53.3086, 67.3487) -> (-53.4824, 67.3837) centre (-53.6044, 66.3291) ccw
  arc A496 (-53.0433, 67.2446) -> (-53.3086, 67.3487) centre (-53.7437, 65.849) ccw
  arc A497 (-52.7884, 67.0901) -> (-53.0433, 67.2446) centre (-53.882, 65.5734) ccw
  arc A498 (-52.562, 66.8976) -> (-52.7884, 67.0901) centre (-53.8748, 65.5834) ccw
  arc A499 (-52.3821, 66.6806) -> (-52.562, 66.8976) centre (-53.6278, 65.8307) ccw
  arc A500 (-52.3821, 66.6806) -> (-52.3573, 66.6463) centre (-51.7286, 67.1265) ccw
  arc A501 (-52.3573, 66.6463) -> (-52.3339, 66.6182) centre (-52.0112, 66.9106) ccw
  arc A502 (-52.3339, 66.6182) -> (-52.3138, 66.5974) centre (-52.0055, 66.9158) ccw
  arc A503 (-52.3138, 66.5974) -> (-52.3051, 66.5957) centre (-52.3081, 66.6034) ccw
  arc A504 (-52.3051, 66.5957) -> (-52.2805, 66.611) centre (-52.3319, 66.6658) ccw
  arc A505 (-52.2805, 66.611) -> (-51.9201, 66.9494) centre (-549.7167, 596.8155) ccw
  arc A506 (-51.9201, 66.9494) -> (-51.555, 67.2925) centre (-1015.4894, 1092.5952) ccw
  arc A507 (-51.555, 67.2925) -> (-51.5493, 67.3057) centre (-51.5674, 67.3057) ccw
  arc A508 (-51.5493, 67.3057) -> (-51.5511, 67.3111) centre (-51.5584, 67.3057) ccw
  arc A509 (-51.5511, 67.3111) -> (-51.577, 67.3459) centre (-57.6783, 62.7919) ccw
  arc A510 (-51.577, 67.3459) -> (-51.6073, 67.3859) centre (-53.704, 65.7583) ccw
  arc A511 (-51.6073, 67.3859) -> (-51.6434, 67.4317) centre (-55.4356, 64.4141) ccw
  arc A512 (-51.6434, 67.4317) -> (-51.8307, 67.6391) centre (-53.3886, 66.043) ccw
  arc A513 (-51.8307, 67.6391) -> (-52.0622, 67.8451) centre (-54.1816, 65.2306) ccw
  arc A514 (-52.0622, 67.8451) -> (-52.3124, 68.0294) centre (-54.1914, 65.2185) ccw
  arc A515 (-52.3124, 68.0294) -> (-52.556, 68.1715) centre (-53.5902, 66.1179) ccw
  arc A516 (-52.556, 68.1715) -> (-52.7128, 68.2408) centre (-53.319, 66.6563) ccw
  arc A517 (-52.7128, 68.2408) -> (-52.9166, 68.3129) centre (-54.2275, 64.282) ccw
  arc A518 (-52.9166, 68.3129) -> (-53.1248, 68.3747) centre (-54.2334, 64.2639) ccw
  arc A519 (-53.1248, 68.3747) -> (-53.2958, 68.4121) centre (-53.5964, 66.626) ccw
  arc A520 (-53.2958, 68.4121) -> (-53.4493, 68.4322) centre (-53.6461, 66.331) ccw
  arc A521 (-53.4493, 68.4322) -> (-53.6452, 68.4469) centre (-53.9515, 63.0687) ccw
  arc A522 (-53.6452, 68.4469) -> (-53.8342, 68.4544) centre (-53.9543, 63.0201) ccw
  arc A523 (-53.8342, 68.4544) -> (-53.9566, 68.4497) centre (-53.8567, 67.4354) ccw
  arc A524 (-53.9849, 66.7348) -> (-54.24, 66.6166) centre (-53.7509, 65.8954) ccw
  arc A525 (-54.24, 66.6166) -> (-54.4464, 66.4226) centre (-53.7367, 65.8744) ccw
  arc A526 (-54.4464, 66.4226) -> (-54.5806, 66.1757) centre (-53.7487, 65.8837) ccw
  arc A527 (-54.5806, 66.1757) -> (-54.6266, 65.9041) centre (-53.8116, 65.9057) ccw
  arc A528 (-54.6266, 65.9041) -> (-54.5386, 65.5295) centre (-53.7788, 65.9058) ccw
  arc A529 (-54.5386, 65.5295) -> (-54.2936, 65.2285) centre (-53.7535, 65.9183) ccw
  arc A530 (-54.2936, 65.2285) -> (-53.9441, 65.0643) centre (-53.7598, 65.9102) ccw
  arc A531 (-53.9441, 65.0643) -> (-53.5637, 65.0719) centre (-53.77, 65.8637) ccw
  arc A532 (-53.5637, 65.0719) -> (-53.3439, 65.1598) centre (-53.8025, 65.9887) ccw
  arc A533 (-53.3439, 65.1598) -> (-53.1618, 65.2969) centre (-53.7393, 65.8743) ccw
  arc A534 (-53.1618, 65.2969) -> (-53.0247, 65.479) centre (-53.7393, 65.8743) ccw
  arc A535 (-53.0247, 65.479) -> (-52.9369, 65.6988) centre (-53.8536, 65.9376) ccw
  arc A536 (-52.9369, 65.6988) -> (-52.9297, 66.0834) centre (-53.733, 65.9062) ccw
  arc A537 (-52.9297, 66.0834) -> (-53.0974, 66.4344) centre (-53.7672, 65.8986) ccw
  arc A538 (-53.0974, 66.4344) -> (-53.4045, 66.6773) centre (-53.7775, 65.8904) ccw
  arc A539 (-53.4045, 66.6773) -> (-53.7859, 66.7602) centre (-53.7732, 65.8996) ccw
  arc A540 (-53.7859, 66.7602) -> (-53.8358, 66.7578) centre (-53.7746, 65.9967) ccw
  arc A541 (-53.8358, 66.7578) -> (-53.8914, 66.7521) centre (-53.7396, 65.5614) ccw
  arc A542 (-53.8914, 66.7521) -> (-53.9443, 66.7441) centre (-53.7479, 65.6266) ccw
  arc A543 (-53.9443, 66.7441) -> (-53.9849, 66.7348) centre (-53.8705, 66.3245) ccw
  arc A544 (-9.2413, 17.0805) -> (-8.2836, 17.2367) centre (-9.779, 23.3947) ccw
  arc A545 (-8.2836, 17.2367) -> (-7.3719, 17.5362) centre (-9.7146, 23.1295) ccw
  arc A546 (-7.3719, 17.5362) -> (-6.5197, 17.9755) centre (-9.7102, 23.1189) ccw
  arc A547 (-6.5197, 17.9755) -> (-5.739, 18.5475) centre (-9.8311, 23.3138) ccw
  arc A548 (-5.739, 18.5475) -> (-5.5697, 18.7002) centre (-8.7857, 22.0962) ccw
  arc A549 (-5.5697, 18.7002) -> (-5.3756, 18.8894) centre (-11.9553, 25.4432) ccw
  arc A550 (-5.3756, 18.8894) -> (-5.1963, 19.0746) centre (-11.7977, 25.2861) ccw
  arc A551 (-5.1963, 19.0746) -> (-5.0811, 19.2079) centre (-6.7042, 20.4934) ccw
  line L81 (-5.0811, 19.2079) -> (-5.0236, 19.2806)
  line L82 (-5.0236, 19.2806) -> (-5.4049, 19.6316)
  line L83 (-5.4049, 19.6316) -> (-5.7862, 19.9826)
  line L84 (-5.7862, 19.9826) -> (-5.8882, 19.8662)
  arc A552 (-6.4861, 19.284) -> (-5.8882, 19.8662) centre (-9.8321, 23.3187) ccw
  arc A553 (-7.1692, 18.8037) -> (-6.4861, 19.284) centre (-9.8382, 23.3261) ccw
  arc A554 (-7.9131, 18.4418) -> (-7.1692, 18.8037) centre (-9.7889, 23.2424) ccw
  arc A555 (-8.6921, 18.2113) -> (-7.9131, 18.4418) centre (-9.6579, 22.9072) ccw
  arc A556 (-9.2057, 18.1331) -> (-8.6921, 18.2113) centre (-9.7026, 23.1248) ccw
  arc A557 (-9.7322, 18.107) -> (-9.2057, 18.1331) centre (-9.7322, 23.4223) ccw
  arc A558 (-10.2587, 18.1331) -> (-9.7322, 18.107) centre (-9.7322, 23.4223) ccw
  arc A559 (-10.7723, 18.2113) -> (-10.2587, 18.1331) centre (-9.7618, 23.1248) ccw
  arc A560 (-11.5514, 18.4415) -> (-10.7723, 18.2113) centre (-9.8024, 22.9274) ccw
  arc A561 (-12.2933, 18.8021) -> (-11.5514, 18.4415) centre (-9.6926, 23.2091) ccw
  arc A562 (-12.9753, 19.2818) -> (-12.2933, 18.8021) centre (-9.6355, 23.3058) ccw
  arc A563 (-13.5761, 19.866) -> (-12.9753, 19.2818) centre (-9.5677, 23.3875) ccw
  line L85 (-13.5761, 19.866) -> (-13.6782, 19.9822)
  line L86 (-13.6782, 19.9822) -> (-14.0597, 19.6316)
  line L87 (-14.0597, 19.6316) -> (-14.4412, 19.281)
  line L88 (-14.4412, 19.281) -> (-14.3813, 19.2039)
  arc A564 (-14.3813, 19.2039) -> (-14.2565, 19.0613) centre (-13.1217, 20.1812) ccw
  arc A565 (-14.2565, 19.0613) -> (-14.0092, 18.8162) centre (-3.0498, 30.1206) ccw
  arc A566 (-14.0092, 18.8162) -> (-13.7512, 18.5722) centre (-4.0248, 29.1148) ccw
  arc A567 (-13.7512, 18.5722) -> (-13.5649, 18.4124) centre (-11.4359, 21.0818) ccw
  arc A568 (-13.5649, 18.4124) -> (-12.802, 17.8903) centre (-9.6207, 23.3578) ccw
  arc A569 (-12.802, 17.8903) -> (-11.9788, 17.4911) centre (-9.7509, 23.134) ccw
  arc A570 (-11.9788, 17.4911) -> (-11.1041, 17.2199) centre (-9.7456, 23.1473) ccw
  arc A571 (-11.1041, 17.2199) -> (-10.1873, 17.0788) centre (-9.6755, 23.4534) ccw
  arc A572 (-10.1873, 17.0788) -> (-9.9643, 17.0663) centre (-9.8159, 21.705) ccw
  arc A573 (-9.9643, 17.0663) -> (-9.7128, 17.0625) centre (-9.7263, 24.5042) ccw
  arc A574 (-9.7128, 17.0625) -> (-9.4621, 17.0672) centre (-9.7263, 24.4713) ccw
  arc A575 (-9.4621, 17.0672) -> (-9.2413, 17.0805) centre (-9.6221, 21.5521) ccw
  arc A576 (-9.2413, 18.7794) -> (-8.6534, 18.889) centre (-9.815, 23.4902) ccw
  arc A577 (-8.6534, 18.889) -> (-8.0956, 19.0702) centre (-9.7279, 23.145) ccw
  arc A578 (-8.0956, 19.0702) -> (-7.5656, 19.3247) centre (-9.7361, 23.1656) ccw
  arc A579 (-7.5656, 19.3247) -> (-7.0606, 19.6529) centre (-9.9548, 23.5525) ccw
  arc A580 (-7.0606, 19.6529) -> (-6.8979, 19.7869) centre (-8.3094, 21.3355) ccw
  arc A581 (-6.8979, 19.7869) -> (-6.6506, 20.0183) centre (-15.5728, 29.3042) ccw
  arc A582 (-6.6506, 20.0183) -> (-6.4104, 20.2542) centre (-17.3207, 31.1235) ccw
  arc A583 (-6.4104, 20.2542) -> (-6.311, 20.3732) centre (-7.0395, 20.8809) ccw
  line L89 (-6.311, 20.3732) -> (-6.2712, 20.4303)
  line L90 (-6.2712, 20.4303) -> (-6.6497, 20.7876)
  line L91 (-6.6497, 20.7876) -> (-7.0281, 21.1449)
  line L92 (-7.0281, 21.1449) -> (-7.1055, 21.0515)
  arc A584 (-7.42, 20.7158) -> (-7.1055, 21.0515) centre (-10.0062, 23.4538) ccw
  arc A585 (-7.7658, 20.4297) -> (-7.42, 20.7158) centre (-9.7629, 23.1961) ccw
  arc A586 (-8.1409, 20.1954) -> (-7.7658, 20.4297) centre (-9.7034, 23.1138) ccw
  arc A587 (-8.5428, 20.014) -> (-8.1409, 20.1954) centre (-9.6846, 23.0787) ccw
  arc A588 (-9.5743, 19.8012) -> (-8.5428, 20.014) centre (-9.7473, 23.247) ccw
  arc A589 (-10.6109, 19.9132) -> (-9.5743, 19.8012) centre (-9.7407, 23.1144) ccw
  arc A590 (-11.5656, 20.3424) -> (-10.6109, 19.9132) centre (-9.7333, 23.1418) ccw
  arc A591 (-12.3588, 21.0513) -> (-11.5656, 20.3424) centre (-9.6135, 23.3247) ccw
  line L93 (-12.3588, 21.0513) -> (-12.436, 21.1445)
  line L94 (-12.436, 21.1445) -> (-12.8142, 20.787)
  line L95 (-12.8142, 20.787) -> (-13.1923, 20.4294)
  line L96 (-13.1923, 20.4294) -> (-13.1528, 20.3728)
  arc A592 (-13.1528, 20.3728) -> (-13.1252, 20.3384) centre (-12.8824, 20.5615) ccw
  arc A593 (-13.1252, 20.3384) -> (-13.0498, 20.2573) centre (-6.3279, 26.584) ccw
  arc A594 (-13.0498, 20.2573) -> (-12.9584, 20.1617) centre (-6.8687, 26.075) ccw
  arc A595 (-12.9584, 20.1617) -> (-12.8577, 20.0592) centre (-4.4477, 28.4259) ccw
  arc A596 (-12.8577, 20.0592) -> (-12.5717, 19.7931) centre (-9.2726, 23.6258) ccw
  arc A597 (-12.5717, 19.7931) -> (-12.2821, 19.5663) centre (-9.9736, 22.8114) ccw
  arc A598 (-12.2821, 19.5663) -> (-11.9733, 19.3675) centre (-9.9819, 22.7997) ccw
  arc A599 (-11.9733, 19.3675) -> (-11.6297, 19.1857) centre (-9.4749, 23.6737) ccw
  arc A600 (-11.6297, 19.1857) -> (-11.2883, 19.0399) centre (-9.8103, 22.9749) ccw
  arc A601 (-11.2883, 19.0399) -> (-10.9284, 18.9216) centre (-9.686, 23.306) ccw
  arc A602 (-10.9284, 18.9216) -> (-10.5594, 18.8334) centre (-9.6828, 23.3174) ccw
  arc A603 (-10.5594, 18.8334) -> (-10.1908, 18.7779) centre (-9.742, 23.0144) ccw
  arc A604 (-10.1908, 18.7779) -> (-9.9934, 18.7649) centre (-9.929, 21.2498) ccw
  arc A605 (-9.9934, 18.7649) -> (-9.7075, 18.7614) centre (-9.7234, 29.1694) ccw
  arc A606 (-9.7075, 18.7614) -> (-9.4242, 18.7657) centre (-9.7237, 29.3221) ccw
  arc A607 (-9.4242, 18.7657) -> (-9.2413, 18.7794) centre (-9.4803, 20.7415) ccw
  arc A608 (-9.5434, 20.4503) -> (-9.0552, 20.5352) centre (-9.8712, 23.7792) ccw
  arc A609 (-9.0552, 20.5352) -> (-8.6122, 20.6889) centre (-9.7096, 23.1369) ccw
  arc A610 (-8.6122, 20.6889) -> (-8.2116, 20.9135) centre (-9.6623, 23.0313) ccw
  arc A611 (-8.2116, 20.9135) -> (-7.8493, 21.2097) centre (-9.7746, 23.1952) ccw
  arc A612 (-7.8493, 21.2097) -> (-7.7329, 21.3272) centre (-10.6671, 24.1156) ccw
  arc A613 (-7.7329, 21.3272) -> (-7.622, 21.4489) centre (-10.618, 24.069) ccw
  arc A614 (-7.622, 21.4489) -> (-7.5253, 21.5617) centre (-13.3375, 26.4473) ccw
  arc A615 (-7.5253, 21.5617) -> (-7.5138, 21.5934) centre (-7.563, 21.5934) ccw
  arc A616 (-7.5138, 21.5934) -> (-7.5197, 21.607) centre (-7.5325, 21.5934) ccw
  arc A617 (-7.5197, 21.607) -> (-7.884, 21.95) centre (-910.3811, -936.9121) ccw
  arc A618 (-7.884, 21.95) -> (-8.2435, 22.2882) centre (-469.987, -469.0133) ccw
  arc A619 (-8.2435, 22.2882) -> (-8.2689, 22.3041) centre (-8.2969, 22.2313) ccw
  arc A620 (-8.2689, 22.3041) -> (-8.2777, 22.3021) centre (-8.2718, 22.2966) ccw
  arc A621 (-8.2777, 22.3021) -> (-8.3041, 22.2731) centre (-7.5009, 21.5676) ccw
  arc A622 (-8.3041, 22.2731) -> (-8.3348, 22.236) centre (-7.7116, 21.7527) ccw
  arc A623 (-8.3348, 22.236) -> (-8.3684, 22.1908) centre (-7.1758, 21.3372) ccw
  arc A624 (-8.5704, 21.9586) -> (-8.3684, 22.1908) centre (-9.6953, 23.1405) ccw
  arc A625 (-8.8146, 21.7653) -> (-8.5704, 21.9586) centre (-9.7506, 23.1987) ccw
  arc A626 (-9.0914, 21.6184) -> (-8.8146, 21.7653) centre (-9.7618, 23.2158) ccw
  arc A627 (-9.3897, 21.524) -> (-9.0914, 21.6184) centre (-9.7586, 23.2082) ccw
  arc A628 (-9.5647, 21.5009) -> (-9.3897, 21.524) centre (-9.6138, 22.5471) ccw
  arc A629 (-9.7914, 21.4994) -> (-9.5647, 21.5009) centre (-9.6959, 24.2957) ccw
  arc A630 (-10.0176, 21.5163) -> (-9.7914, 21.4994) centre (-9.6958, 24.2978) ccw
  arc A631 (-10.1914, 21.5513) -> (-10.0176, 21.5163) centre (-9.8956, 22.5709) ccw
  arc A632 (-10.4567, 21.6554) -> (-10.1914, 21.5513) centre (-9.7563, 23.051) ccw
  arc A633 (-10.7116, 21.8099) -> (-10.4567, 21.6554) centre (-9.618, 23.3266) ccw
  arc A634 (-10.938, 22.0024) -> (-10.7116, 21.8099) centre (-9.6252, 23.3166) ccw
  arc A635 (-11.1179, 22.2194) -> (-10.938, 22.0024) centre (-9.8722, 23.0693) ccw
  arc A636 (-11.1179, 22.2194) -> (-11.1427, 22.2537) centre (-11.7714, 21.7735) ccw
  arc A637 (-11.1427, 22.2537) -> (-11.1661, 22.2818) centre (-11.4888, 21.9894) ccw
  arc A638 (-11.1661, 22.2818) -> (-11.1862, 22.3026) centre (-11.4945, 21.9842) ccw
  arc A639 (-11.1862, 22.3026) -> (-11.1949, 22.3043) centre (-11.1919, 22.2966) ccw
  arc A640 (-11.1949, 22.3043) -> (-11.2195, 22.289) centre (-11.1681, 22.2342) ccw
  arc A641 (-11.2195, 22.289) -> (-11.5799, 21.9506) centre (486.2167, -507.9155) ccw
  arc A642 (-11.5799, 21.9506) -> (-11.945, 21.6075) centre (951.9894, -1003.6952) ccw
  arc A643 (-11.945, 21.6075) -> (-11.9507, 21.5943) centre (-11.9326, 21.5943) ccw
  arc A644 (-11.9507, 21.5943) -> (-11.9489, 21.5889) centre (-11.9416, 21.5943) ccw
  arc A645 (-11.9489, 21.5889) -> (-11.923, 21.5541) centre (-5.8217, 26.1081) ccw
  arc A646 (-11.923, 21.5541) -> (-11.8927, 21.5141) centre (-9.796, 23.1417) ccw
  arc A647 (-11.8927, 21.5141) -> (-11.8566, 21.4683) centre (-8.0644, 24.4859) ccw
  arc A648 (-11.8566, 21.4683) -> (-11.6693, 21.2609) centre (-10.1114, 22.857) ccw
  arc A649 (-11.6693, 21.2609) -> (-11.4378, 21.0549) centre (-9.3184, 23.6694) ccw
  arc A650 (-11.4378, 21.0549) -> (-11.1876, 20.8706) centre (-9.3086, 23.6815) ccw
  arc A651 (-11.1876, 20.8706) -> (-10.944, 20.7285) centre (-9.9098, 22.7821) ccw
  arc A652 (-10.944, 20.7285) -> (-10.7872, 20.6592) centre (-10.181, 22.2437) ccw
  arc A653 (-10.7872, 20.6592) -> (-10.5834, 20.5871) centre (-9.2725, 24.618) ccw
  arc A654 (-10.5834, 20.5871) -> (-10.3752, 20.5253) centre (-9.2666, 24.6361) ccw
  arc A655 (-10.3752, 20.5253) -> (-10.2042, 20.4879) centre (-9.9036, 22.274) ccw
  arc A656 (-10.2042, 20.4879) -> (-10.0507, 20.4678) centre (-9.8539, 22.569) ccw
  arc A657 (-10.0507, 20.4678) -> (-9.8548, 20.4531) centre (-9.5485, 25.8313) ccw
  arc A658 (-9.8548, 20.4531) -> (-9.6658, 20.4456) centre (-9.5457, 25.8799) ccw
  arc A659 (-9.6658, 20.4456) -> (-9.5434, 20.4503) centre (-9.6433, 21.4646) ccw
  arc A660 (-9.5151, 22.1652) -> (-9.26, 22.2834) centre (-9.7491, 23.0046) ccw
  arc A661 (-9.26, 22.2834) -> (-9.0536, 22.4774) centre (-9.7633, 23.0256) ccw
  arc A662 (-9.0536, 22.4774) -> (-8.9194, 22.7243) centre (-9.7513, 23.0163) ccw
  arc A663 (-8.9194, 22.7243) -> (-8.8734, 22.9959) centre (-9.6884, 22.9943) ccw
  arc A664 (-8.8734, 22.9959) -> (-8.9614, 23.3705) centre (-9.7212, 22.9942) ccw
  arc A665 (-8.9614, 23.3705) -> (-9.2064, 23.6715) centre (-9.7465, 22.9817) ccw
  arc A666 (-9.2064, 23.6715) -> (-9.5559, 23.8357) centre (-9.7402, 22.9898) ccw
  arc A667 (-9.5559, 23.8357) -> (-9.9363, 23.8281) centre (-9.73, 23.0363) ccw
  arc A668 (-9.9363, 23.8281) -> (-10.1561, 23.7402) centre (-9.6975, 22.9113) ccw
  arc A669 (-10.1561, 23.7402) -> (-10.3382, 23.6031) centre (-9.7607, 23.0257) ccw
  arc A670 (-10.3382, 23.6031) -> (-10.4753, 23.421) centre (-9.7607, 23.0257) ccw
  arc A671 (-10.4753, 23.421) -> (-10.5631, 23.2012) centre (-9.6464, 22.9624) ccw
  arc A672 (-10.5631, 23.2012) -> (-10.5703, 22.8166) centre (-9.767, 22.9938) ccw
  arc A673 (-10.5703, 22.8166) -> (-10.4026, 22.4656) centre (-9.7328, 23.0014) ccw
  arc A674 (-10.4026, 22.4656) -> (-10.0955, 22.2227) centre (-9.7225, 23.0096) ccw
  arc A675 (-10.0955, 22.2227) -> (-9.7141, 22.1398) centre (-9.7268, 23.0004) ccw
  arc A676 (-9.7141, 22.1398) -> (-9.6642, 22.1422) centre (-9.7254, 22.9033) ccw
  arc A677 (-9.6642, 22.1422) -> (-9.6086, 22.1479) centre (-9.7604, 23.3386) ccw
  arc A678 (-9.6086, 22.1479) -> (-9.5557, 22.1559) centre (-9.7521, 23.2734) ccw
  arc A679 (-9.5557, 22.1559) -> (-9.5151, 22.1652) centre (-9.6295, 22.5755) ccw
  line L97 (-50.5534, 75.3641) -> (-56.819, 75.3641)
  line L98 (-56.819, 75.3641) -> (-56.819, 76.8049)
  spline S0 degree 2 poles (-56.819, 76.8049) (-56.1439, 77.4389) (-54.9418, 78.6163) (-54.3654, 79.2502) knots 0 0 0 1 2 2 2
  spline S1 degree 2 poles (-54.3654, 79.2502) (-53.2045, 80.5264) (-52.3565, 82.0578) (-52.3565, 82.8729) knots 0 0 0 1 2 2 2
  spline S2 degree 2 poles (-52.3565, 82.8729) (-52.3565, 83.3011) (-52.62, 83.9433) (-52.8587, 84.1491) knots 0 0 0 1 2 2 2
  spline S3 degree 2 poles (-52.8587, 84.1491) (-53.0975, 84.3549) (-53.7232, 84.5608) (-54.102, 84.5608) knots 0 0 0 1 2 2 2
  spline S4 degree 2 poles (-54.102, 84.5608) (-54.4642, 84.5608) (-55.2052, 84.3796) (-55.5428, 84.2397) knots 0 0 0 1 2 2 2
  spline S5 degree 2 poles (-55.5428, 84.2397) (-55.831, 84.1244) (-56.3662, 83.7951) (-56.5308, 83.6798) knots 0 0 0 1 2 2 2
  line L99 (-56.5308, 83.6798) -> (-56.6049, 83.6798)
  line L100 (-56.6049, 83.6798) -> (-56.6049, 85.1289)
  spline S6 degree 2 poles (-56.6049, 85.1289) (-56.185, 85.3347) (-54.6783, 85.7381) (-54.0032, 85.7381) knots 0 0 0 1 2 2 2
  spline S7 degree 2 poles (-54.0032, 85.7381) (-52.5788, 85.7381) (-50.9733, 84.2314) (-50.9733, 82.947) knots 0 0 0 1 2 2 2
  spline S8 degree 2 poles (-50.9733, 82.947) (-50.9733, 82.346) (-51.2532, 81.3415) (-51.5002, 80.9134) knots 0 0 0 1 2 2 2
  spline S9 degree 2 poles (-51.5002, 80.9134) (-51.7472, 80.4688) (-52.4635, 79.596) (-52.8587, 79.1761) knots 0 0 0 1 2 2 2
  spline S10 degree 2 poles (-52.8587, 79.1761) (-53.5009, 78.4763) (-55.0735, 76.9778) (-55.5428, 76.5415) knots 0 0 0 1 2 2 2
  line L101 (-55.5428, 76.5415) -> (-50.5534, 76.5415)
  line L102 (-50.5534, 76.5415) -> (-50.5534, 75.3641)
  line L103 (-12.9466, 13.8805) -> (-6.681, 13.8805)
  line L104 (-6.681, 13.8805) -> (-6.681, 12.4397)
  spline S11 degree 2 poles (-6.681, 12.4397) (-7.3561, 11.8057) (-8.5582, 10.6283) (-9.1346, 9.9943) knots 0 0 0 1 2 2 2
  spline S12 degree 2 poles (-9.1346, 9.9943) (-10.2955, 8.7182) (-11.1435, 7.1868) (-11.1435, 6.3716) knots 0 0 0 1 2 2 2
  spline S13 degree 2 poles (-11.1435, 6.3716) (-11.1435, 5.9435) (-10.88, 5.3013) (-10.6413, 5.0955) knots 0 0 0 1 2 2 2
  spline S14 degree 2 poles (-10.6413, 5.0955) (-10.4025, 4.8896) (-9.7768, 4.6838) (-9.398, 4.6838) knots 0 0 0 1 2 2 2
  spline S15 degree 2 poles (-9.398, 4.6838) (-9.0358, 4.6838) (-8.2948, 4.8649) (-7.9572, 5.0049) knots 0 0 0 1 2 2 2
  spline S16 degree 2 poles (-7.9572, 5.0049) (-7.669, 5.1202) (-7.1338, 5.4495) (-6.9692, 5.5648) knots 0 0 0 1 2 2 2
  line L105 (-6.9692, 5.5648) -> (-6.8951, 5.5648)
  line L106 (-6.8951, 5.5648) -> (-6.8951, 4.1157)
  spline S17 degree 2 poles (-6.8951, 4.1157) (-7.315, 3.9099) (-8.8217, 3.5064) (-9.4968, 3.5064) knots 0 0 0 1 2 2 2
  spline S18 degree 2 poles (-9.4968, 3.5064) (-10.9212, 3.5064) (-12.5267, 5.0131) (-12.5267, 6.2975) knots 0 0 0 1 2 2 2
  spline S19 degree 2 poles (-12.5267, 6.2975) (-12.5267, 6.8986) (-12.2468, 7.9031) (-11.9998, 8.3312) knots 0 0 0 1 2 2 2
  spline S20 degree 2 poles (-11.9998, 8.3312) (-11.7528, 8.7758) (-11.0365, 9.6485) (-10.6413, 10.0684) knots 0 0 0 1 2 2 2
  spline S21 degree 2 poles (-10.6413, 10.0684) (-9.9991, 10.7683) (-8.4265, 12.2668) (-7.9572, 12.7031) knots 0 0 0 1 2 2 2
  line L107 (-7.9572, 12.7031) -> (-12.9466, 12.7031)
  line L108 (-12.9466, 12.7031) -> (-12.9466, 13.8805)
  line L109 (-50.5534, 75.3641) -> (-56.819, 75.3641)
  line L110 (-56.819, 75.3641) -> (-56.819, 76.8049)
  spline S22 degree 2 poles (-56.819, 76.8049) (-56.1439, 77.4389) (-54.9418, 78.6163) (-54.3654, 79.2502) knots 0 0 0 1 2 2 2
  spline S23 degree 2 poles (-54.3654, 79.2502) (-53.2045, 80.5264) (-52.3565, 82.0578) (-52.3565, 82.8729) knots 0 0 0 1 2 2 2
  spline S24 degree 2 poles (-52.3565, 82.8729) (-52.3565, 83.3011) (-52.62, 83.9433) (-52.8587, 84.1491) knots 0 0 0 1 2 2 2
  spline S25 degree 2 poles (-52.8587, 84.1491) (-53.0975, 84.3549) (-53.7232, 84.5608) (-54.102, 84.5608) knots 0 0 0 1 2 2 2
  spline S26 degree 2 poles (-54.102, 84.5608) (-54.4642, 84.5608) (-55.2052, 84.3796) (-55.5428, 84.2397) knots 0 0 0 1 2 2 2
  spline S27 degree 2 poles (-55.5428, 84.2397) (-55.831, 84.1244) (-56.3662, 83.7951) (-56.5308, 83.6798) knots 0 0 0 1 2 2 2
  line L111 (-56.5308, 83.6798) -> (-56.6049, 83.6798)
  line L112 (-56.6049, 83.6798) -> (-56.6049, 85.1289)
  spline S28 degree 2 poles (-56.6049, 85.1289) (-56.185, 85.3347) (-54.6783, 85.7381) (-54.0032, 85.7381) knots 0 0 0 1 2 2 2